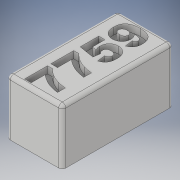
# Autodesk Inventor part: 7759Block
Saved by Autodesk Inventor 2019 (Build 230136000, 136)
## iProperties
Created: 2019-10-29
Part Number: 7759Block
Material: Generic
Document SubType Name: Modeling
Designer: james
Density: 1 g/cm^3
Appearance: Default
Author: james
Autodesk Inventor part; units mm, degrees
ref_plane "YZ Plane" through (0, 0, 0) normal (1, 0, 0) x (0, 1, 0)
ref_plane "XZ Plane" through (0, 0, 0) normal (0, 1, 0) x (-1, 0, 0)
ref_plane "XY Plane" through (0, 0, 0) normal (0, 0, 1) x (1, 0, 0)
sketch "Sketch1" plane through (0, 0, 0) normal (0, 1, 0) x (-1, 0, 0)
  line L0 (65.2374, 90.5054) -> (-34.7626, 90.5054)
  line L1 (-34.7626, 90.5054) -> (-34.7626, -109.4946)
  line L2 (-34.7626, -109.4946) -> (65.2374, -109.4946)
  line L3 (65.2374, -109.4946) -> (65.2374, 90.5054)
  point P0 (0, 0)
  dimension "d0" = 200
  dimension "d1" = 100
  constraints: 8 end point, 2 parallel, 1 horizontal, 1 perpendicular
  measures "d0" distance of L0.end L1.end
  measures "d1" distance of L1.end L2.end
extrude "Extrusion1" add sketch "Sketch1" along normal blind 100
sketch "Sketch2" plane through (0, 0, 0) normal (0, -1, 0) x (1, 0, 0)
  line L0 (17.7626, 73.5054) -> (-48.2374, 73.5054)
  line L1 (-48.2374, 73.5054) -> (-48.2374, -92.4946)
  line L2 (-48.2374, -92.4946) -> (17.7626, -92.4946)
  line L3 (17.7626, -92.4946) -> (17.7626, 73.5054)
  line L4 (34.7626, 90.5054) -> (34.7626, -109.4946) projected
  line L5 (-65.2374, 90.5054) -> (34.7626, 90.5054) projected
  line L6 (34.7626, -109.4946) -> (-65.2374, -109.4946) projected
  line L7 (-65.2374, -109.4946) -> (-65.2374, 90.5054) projected
  point P0 (0, 0)
  dimension "d4" = 17
  dimension "d5" = 17
  dimension "d6" = 17
  dimension "d7" = 17
  constraints: 8 end point, 2 parallel, 1 horizontal, 1 perpendicular
  measures "d4" distance between parallel lines of L3 L4
  measures "d5" distance between parallel lines of L5 L0
  measures "d6" distance between parallel lines of L6 L2
  measures "d7" distance between parallel lines of L7 L1
extrude "Extrusion2" cut sketch "Sketch2" against normal blind 38 contours L3 L2 L1 L0
fillet "Fillet1" radius 6.35 8 edges at (-15.2374, 100, 90.5054) (34.7626, 100, -9.4946) (34.7626, 50, 90.5054) (-65.2374, 50, 90.5054) (-65.2374, 100, -9.4946) (-15.2374, 100, -109.4946) (34.7626, 50, -109.4946) (-65.2374, 50, -109.4946)
sketch "Sketch3" plane through (0, 100, 0) normal (0, 1, 0) x (1, 0, 0)
  line L0 (-42.3145, -85.4273) -> (-42.3145, -16.4468) construction
  line L1 (-42.3145, -16.4468) -> (96.9241, -16.4468) construction
  line L2 (96.9241, -16.4468) -> (96.9241, -85.4273) construction
  line L3 (96.9241, -85.4273) -> (-42.3145, -85.4273) construction
  line L4 (-41.4344, -82.2493) -> (-41.4344, -41.0812)
  line L5 (-41.4344, -41.0812) -> (-31.9002, -41.0812)
  spline S0 degree 2 poles (-31.9002, -41.0812) (-27.0598, -46.4595) (-21.3882, -50.0287) knots 0 0 0 1 1 1
  spline S1 degree 2 poles (-21.3882, -50.0287) (-14.5432, -54.3802) (-6.1335, -56.9226) knots 0 0 0 1 1 1
  spline S2 degree 2 poles (-6.1335, -56.9226) (0.4181, -58.9272) (9.3656, -59.6117) knots 0 0 0 1 1 1
  line L6 (9.3656, -59.6117) -> (9.3656, -73.693)
  spline S3 degree 2 poles (9.3656, -73.693) (-3.0533, -72.0306) (-19.9214, -64.8922) (-29.5045, -57.1671) knots 0 0 0 1 2 2 2
  line L7 (-29.5045, -57.1671) -> (-29.5045, -82.2493)
  line L8 (-29.5045, -82.2493) -> (-41.4344, -82.2493)
  line L9 (-41.4344, -34.8718) -> (-41.4344, 6.2962)
  line L10 (-41.4344, 6.2962) -> (-31.9002, 6.2962)
  spline S4 degree 2 poles (-31.9002, 6.2962) (-27.0598, 0.918) (-21.3882, -2.6512) knots 0 0 0 1 1 1
  spline S5 degree 2 poles (-21.3882, -2.6512) (-14.5432, -7.0027) (-6.1335, -9.5451) knots 0 0 0 1 1 1
  spline S6 degree 2 poles (-6.1335, -9.5451) (0.4181, -11.5498) (9.3656, -12.2343) knots 0 0 0 1 1 1
  line L11 (9.3656, -12.2343) -> (9.3656, -26.3155)
  spline S7 degree 2 poles (9.3656, -26.3155) (-3.0533, -24.6531) (-19.9214, -17.5147) (-29.5045, -9.7896) knots 0 0 0 1 2 2 2
  line L12 (-29.5045, -9.7896) -> (-29.5045, -34.8718)
  line L13 (-29.5045, -34.8718) -> (-41.4344, -34.8718)
  line L14 (-41.4344, 17.9817) -> (-41.4344, 51.4246)
  line L15 (-41.4344, 51.4246) -> (-30.189, 51.4246)
  line L16 (-30.189, 51.4246) -> (-30.189, 28.7871)
  line L17 (-30.189, 28.7871) -> (-22.5616, 27.6137)
  spline S8 degree 2 poles (-22.5616, 27.6137) (-23.6373, 29.9605) (-24.7618, 34.5565) (-24.7618, 36.8056) knots 0 0 0 1 2 2 2
  spline S9 degree 2 poles (-24.7618, 36.8056) (-24.7618, 44.384) (-15.521, 53.8693) (-8.5293, 53.8693) knots 0 0 0 1 2 2 2
  spline S10 degree 2 poles (-8.5293, 53.8693) (-3.64, 53.8693) (5.4541, 48.98) (10.2457, 40.0325) (10.2457, 33.0408) knots 0 0 0 1 2 3 3 3
  spline S11 degree 2 poles (10.2457, 33.0408) (10.2457, 28.0048) (8.3388, 20.8664) (4.5741, 15.8304) (-0.2175, 12.7012) (-3.7867, 11.6745) knots 0 0 0 1 2 3 4 4 4
  line L18 (-3.7867, 11.6745) -> (-5.3512, 25.9513)
  spline S12 degree 2 poles (-5.3512, 25.9513) (-1.9287, 26.4891) (1.6405, 30.2539) (1.6405, 32.8941) knots 0 0 0 1 2 2 2
  spline S13 degree 2 poles (1.6405, 32.8941) (1.6405, 35.8277) (-2.8088, 39.6414) (-7.2581, 39.6414) knots 0 0 0 1 2 2 2
  spline S14 degree 2 poles (-7.2581, 39.6414) (-11.8051, 39.6414) (-16.01, 35.7788) (-16.01, 32.6008) knots 0 0 0 1 2 2 2
  spline S15 degree 2 poles (-16.01, 32.6008) (-16.01, 30.5473) (-14.9832, 28.6404) knots 0 0 0 1 1 1
  spline S16 degree 2 poles (-14.9832, 28.6404) (-14.2987, 27.2714) (-12.3919, 25.5601) knots 0 0 0 1 1 1
  line L19 (-12.3919, 25.5601) -> (-14.1031, 13.5324)
  line L20 (-14.1031, 13.5324) -> (-41.4344, 17.9817)
  line L21 (-2.0265, 60.2254) -> (-3.7867, 74.2577)
  spline S17 degree 2 poles (-3.7867, 74.2577) (-0.8531, 74.7956) (1.5916, 77.4358) (1.5916, 79.3426) knots 0 0 0 1 2 2 2
  spline S18 degree 2 poles (1.5916, 79.3426) (1.5916, 82.7652) (-1.8309, 84.672) knots 0 0 0 1 1 1
  spline S19 degree 2 poles (-1.8309, 84.672) (-4.3734, 86.041) (-12.5874, 86.7255) knots 0 0 0 1 1 1
  spline S20 degree 2 poles (-12.5874, 86.7255) (-9.9961, 84.1831) (-7.5514, 78.8537) (-7.5514, 75.3823) knots 0 0 0 1 2 2 2
  spline S21 degree 2 poles (-7.5514, 75.3823) (-7.5514, 68.5372) (-17.2323, 59.1498) (-24.664, 59.1498) knots 0 0 0 1 2 2 2
  spline S22 degree 2 poles (-24.664, 59.1498) (-29.7489, 59.1498) (-38.0608, 63.9413) (-42.3145, 72.302) (-42.3145, 78.6581) knots 0 0 0 1 2 3 3 3
  spline S23 degree 2 poles (-42.3145, 78.6581) (-42.3145, 86.2855) (-37.0829, 95.4774) (-25.6908, 101.0023) (-16.3033, 101.0023) knots 0 0 0 1 2 3 3 3
  spline S24 degree 2 poles (-16.3033, 101.0023) (-2.5643, 101.0023) (10.2457, 89.4146) (10.2457, 79.196) knots 0 0 0 1 2 2 2
  spline S25 degree 2 poles (10.2457, 79.196) (10.2457, 73.1332) (7.4588, 66.0926) (2.0316, 61.4966) (-2.0265, 60.2254) knots 0 0 0 1 2 3 3 3
  spline S26 degree 2 poles (-24.7129, 86.1877) (-28.82, 86.1877) (-33.5137, 82.0318) (-33.5137, 79.0493) knots 0 0 0 1 2 2 2
  spline S27 degree 2 poles (-33.5137, 79.0493) (-33.5137, 76.2624) (-29.3089, 72.5465) (-25.0552, 72.5465) knots 0 0 0 1 2 2 2
  spline S28 degree 2 poles (-25.0552, 72.5465) (-20.8015, 72.5465) (-16.3033, 76.409) (-16.3033, 79.2937) knots 0 0 0 1 2 2 2
  spline S29 degree 2 poles (-16.3033, 79.2937) (-16.3033, 82.2762) (-20.6548, 86.1877) (-24.7129, 86.1877) knots 0 0 0 1 2 2 2
  point P0 (0, 0)
  constraints: 2 other
extrude "Extrusion3" cut sketch "Sketch3" against normal blind 12.8
body "Solid1"
